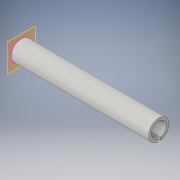
# Autodesk Inventor part: Pickup Pvc
Saved by Autodesk Inventor 2016 (Build 200138000, 138)
## iProperties
Created: 2015-11-25
Part Number: Pickup Pvc
Material: PVC-Piping
Document SubType Name: Modeling
Designer: Julia
Density: 1.4 g/cm^3
Appearance: Smooth - White
Author: Julia
Autodesk Inventor part; units mm, degrees
ref_plane "YZ Plane" through (0, 0, 0) normal (1, 0, 0) x (0, 1, 0)
ref_plane "XZ Plane" through (0, 0, 0) normal (0, 1, 0) x (-1, 0, 0)
ref_plane "XY Plane" through (0, 0, 0) normal (0, 0, 1) x (1, 0, 0)
ref_plane "Work Plane1" through (107.95, 0, 0) normal (1, 0, 0) x (0, 0, -1)
ref_plane "Work Plane2" through (107.95, 0, 0) normal (1, 0, 0) x (0, 0, -1)
sketch "Sketch3" plane through (107.95, 0, 0) normal (1, 0, 0) x (0, 0, -1)
  line L0 (0, 0) -> (0, -8.001)
  circle A0 centre (0, 0) radius 8.001 projected
  line L1 (0, 0) -> (0, -8.001)
  line L2 (0, -8.001) -> (0, 0)
  constraints: 6 end point, 3 vertical, 1 vertical alignment, 1 other
ref_plane "Work Plane3" through (107.95, 0, 0) normal (1, 0, 0) x (0, 0, -1)
sketch "Sketch4" plane through (107.95, 0, 0) normal (1, 0, 0) x (0, 0, -1)
  line L0 (0, 0) -> (1.1557, 0)
  line L1 (0, 0) -> (-1.1557, 0)
  line L2 (1.1557, 0) -> (1.1557, -7.9171)
  circle A0 centre (0, 0) radius 8.001 projected
  line L3 (-1.1557, 0) -> (-1.1557, -7.9171)
  line L4 (-1.1557, -7.9171) -> (1.1557, -7.9171)
  dimension "d6" = 1.1557
  dimension "d7" = 1.1557
  constraints: 10 end point, 2 horizontal, 2 point on circle, 1 parallel, 1 vertical
  measures "d6" distance of L0.start L0.end
  measures "d7" distance of L0.start L1.end
ref_plane "Work Plane4" through (107.95, 0, 0) normal (1, 0, 0) x (0, 0, -1)
sketch "Sketch5" plane through (107.95, 0, 0) normal (1, 0, 0) x (0, 0, -1)
  circle A0 centre (0, 0) radius 8.001 projected
  line L0 (-1.1477, 0) -> (0, 0)
  line L1 (0, 0) -> (0, -8.001)
  line L2 (0, -8.001) -> (-1.1477, -8.001)
  line L3 (-1.1477, -8.001) -> (-1.1477, 0)
  constraints: 8 end point, 2 parallel, 1 horizontal, 1 perpendicular, 1 vertical alignment, 1 other
extrude "Extrusion3" add sketch "Sketch4" along normal blind 107.95 contours L1 L3 A0 L2 L0
sketch "Sketch6" plane through (215.9, 0, 0) normal (1, 0, 0) x (0, 0, -1)
  circle A0 centre (0, 0) radius 5.842
  dimension "d10" = 11.684
  constraints: 1 centre point, 1 coincident
  measures "d10" diameter of A0
extrude "Extrusion4" cut sketch "Sketch6" against normal blind 107.95
body "Solid1"
